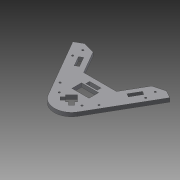
# Autodesk Inventor part: Frame_Upper_Plate_Bottom
Saved by Autodesk Inventor 2014 (Build 180170000, 170)
## iProperties
Created: 2014-08-25
Part Number: Frame_Upper_Plate_Bottom
Material: Generic
Document SubType Name: Modeling
Designer: ThatOtherGuy
Density: 1 g/cm^3
Appearance: Default
Author: ThatOtherGuy
Autodesk Inventor part; units mm, degrees
ref_plane "YZ Plane" through (0, 0, 0) normal (1, 0, 0) x (0, 1, 0)
ref_plane "XZ Plane" through (0, 0, 0) normal (0, 1, 0) x (-1, 0, 0)
ref_plane "XY Plane" through (0, 0, 0) normal (0, 0, 1) x (1, 0, 0)
sketch "Sketch1" plane through (0, 0, 0) normal (0, 0, 1) x (1, 0, 0)
  line L0 (-10.6066, 0) -> (0, 10.6066)
  line L1 (0, 10.6066) -> (10.6066, 0)
  line L2 (10.6066, 0) -> (0, -10.6066)
  line L3 (0, -10.6066) -> (-10.6066, 0)
  arc A0 (-25.9808, -15) -> (25.9808, -15) centre (0, 0) ccw
  line L4 (25.9808, -15) -> (85, 87.2243)
  line L5 (10, 41.731) -> (10, 35)
  line L6 (10, 35) -> (-10, 35)
  line L7 (-10, 35) -> (-10, 41.731)
  line L8 (-10, 41.731) -> (10, 41.731)
  line L9 (-85, 87.2243) -> (-25.9808, -15)
  circle A1 centre (-49.0748, 40) radius 1.6
  circle A2 centre (-64.0748, 65.9808) radius 1.6
  circle A3 centre (49.0748, 40) radius 1.6
  circle A4 centre (64.0748, 65.9808) radius 1.6
  line L10 (-85, 87.2243) -> (-72.0096, 94.7243)
  line L11 (-51.5192, 89.2339) -> (-28.8675, 50)
  line L12 (-28.8675, 50) -> (28.8675, 50)
  line L13 (28.8675, 50) -> (51.5192, 89.2339)
  line L14 (2.6517, -7.955) -> (7.955, -2.6517)
  line L15 (7.955, -2.6517) -> (12.7145, -7.4112)
  line L16 (12.7145, -7.4112) -> (7.4112, -12.7145)
  line L17 (7.4112, -12.7145) -> (2.6517, -7.955)
  line L18 (-2.6517, -7.955) -> (-7.4112, -12.7145)
  line L19 (-7.4112, -12.7145) -> (-12.7145, -7.4112)
  line L20 (-12.7145, -7.4112) -> (-7.955, -2.6517)
  line L21 (-7.955, -2.6517) -> (-2.6517, -7.955)
  circle A5 centre (-38.567, 40) radius 1.6
  circle A6 centre (38.567, 40) radius 1.6
  circle A7 centre (-63.567, 83.3013) radius 1.6
  circle A8 centre (63.567, 83.3013) radius 1.6
  circle A9 centre (-20, -1.6) radius 1.6
  circle A10 centre (20, -1.6) radius 1.6
  line L22 (-57.4526, 69.5109) -> (-47.4526, 52.1904)
  line L23 (-47.4526, 52.1904) -> (-41.6234, 55.5559)
  line L24 (-41.6234, 55.5559) -> (-51.6234, 72.8764)
  line L25 (-51.6234, 72.8764) -> (-57.4526, 69.5109)
  line L26 (47.4526, 52.1904) -> (57.4526, 69.5109)
  line L27 (57.4526, 69.5109) -> (51.6234, 72.8764)
  line L28 (51.6234, 72.8764) -> (41.6234, 55.5559)
  line L29 (41.6234, 55.5559) -> (47.4526, 52.1904)
  line L30 (-15, 32.5) -> (15, 32.5)
  line L31 (15, 32.5) -> (15, 15.6066)
  line L32 (15, 15.6066) -> (-15, 15.6066)
  line L33 (-15, 15.6066) -> (-15, 32.5)
  line L34 (-10.6066, 0) -> (10.6066, 0)
  line L35 (25.9808, -15) -> (0, -60)
  line L36 (0, -60) -> (-25.9808, -15)
  line L37 (85, 87.2243) -> (72.0096, 94.7243)
  circle A11 centre (-34.0748, 14.0192) radius 1.6
  circle A12 centre (34.0748, 14.0192) radius 1.6
  line L38 (72.0096, 94.7243) -> (51.5192, 89.2339)
  line L39 (-51.5192, 89.2339) -> (-72.0096, 94.7243)
  point P0 (0, 0)
  point P1 (0, 35)
  point P2 (0, 32.5)
  dimension "d0" = 15
  dimension "d9" = 30
  dimension "d11" = 6.731
  dimension "d12" = 20
  dimension "d25" = 60
  dimension "d34" = 3.2
  dimension "d36" = 30
  dimension "d38" = 30
  dimension "d40" = 7.5
  dimension "d41" = 7.5
  dimension "d42" = 7.5
  dimension "d43" = 7.5
  dimension "d45" = 40
  dimension "d54" = 50
  dimension "d55" = 0
  dimension "d56" = 0
  dimension "d57" = 7.5
  dimension "d58" = 3.75
  dimension "d63" = 15
  dimension "d64" = 3.2
  dimension "d66" = 50
  dimension "d67" = 15
  dimension "d68" = 15
  dimension "d73" = 20
  dimension "d74" = 15
  dimension "d75" = 15
  dimension "d76" = 15
  dimension "d77" = 15
  dimension "d79" = 35
  dimension "d80" = 2.5
  dimension "d81" = 5
  dimension "d82" = 30
  dimension "d83" = 20
  dimension "d84" = 20
  dimension "d85" = 40
  dimension "d86" = 170
  dimension "d88" = 30
  dimension "d89" = 30
  dimension "d90" = 7.5
  dimension "d91" = 7.5
  dimension "d92" = 135
  dimension "d93" = 30
  dimension "d94" = 45
  dimension "d95" = 15
  constraints: 80 end point, 14 parallel, 13 centre point, 13 equal length, 13 perpendicular, 10 equal radius, 7 horizontal alignment, 4 vertical alignment, 3 horizontal, 3 tangent, 2 collinear, 2 midpoint, 2 point on circle, 1 coincident
  measures "d0" distance of L0.start L0.end
  measures "d9" radius of A0
  measures "d11" distance of L5.start L5.end
  measures "d12" distance of L5.end L6.end
  measures "d25" angle of L9 L4
  measures "d34" diameter of A2
  measures "d36" distance of A1.centre A2.centre
  measures "d38" distance of A4.centre A3.centre
  measures "d40" distance from line of L4 A3.centre
  measures "d41" distance from line of L4 A4.centre
  measures "d42" distance from line of L9 A1.centre
  measures "d43" distance from line of L9 A2.centre
  measures "d45" vertical distance of A1.centre L0.start
  measures "d54" distance from line of point (0, 0) L12
  measures "d55" distance between parallel lines of L2 L14
  measures "d56" distance between parallel lines of L3 L21
  measures "d57" distance of L18.end L19.end
  measures "d58" distance between parallel lines of L2 L18
  measures "d63" distance edge to line of A6 L4
  measures "d64" diameter of A5
  measures "d66" distance of A5.centre A7.centre
  measures "d67" distance edge to line of A7 L9
  measures "d68" distance edge to line of A8 L4
  measures "d73" distance of L27.end L28.end
  measures "d74" distance between parallel lines of L4 L26
  measures "d75" distance between parallel lines of L9 L22
  measures "d76" distance edge to line of A5 L9
  measures "d77" distance from line of L23 A5.centre
  measures "d79" distance from line of point (0, 0) L6
  measures "d80" distance between parallel lines of L6 L30
  measures "d81" distance from line of L0.end L32
  measures "d82" distance of L30.start L30.end
  measures "d83" horizontal distance of A9.centre point (0, 0)
  measures "d84" horizontal distance of A10.centre point (0, 0)
  measures "d85" vertical distance of point (0, 0) A5.centre
  measures "d86" distance of L4.end L35.end
  measures "d88" distance of A11.centre A1.centre
  measures "d89" distance of A3.centre A12.centre
  measures "d90" distance from line of L9 A11.centre
  measures "d91" distance from line of L4 A12.centre
  measures "d92" angle of L10 L39
  measures "d93" distance between parallel lines of L11 L9
  measures "d94" angle of L37 L38
  measures "d95" distance of L9.start L10.end
extrude "Extrusion2" add sketch "Sketch1" along normal blind 6.731 contours L9 L10 L39 L11 L12 L13 L38 L37 L4 A0 | A5 | A6
sketch "Sketch2" plane through (0, 0, 6.731) normal (0, 0, 1) x (1, 0, 0)
  circle A0 centre (49.0748, 40) radius 1.6 projected
  circle A1 centre (-49.0748, 40) radius 1.6 projected
extrude "Extrusion3" add sketch "Sketch2" against normal up to surface (6.731 mm away)
equation "\"d38\" = d36"
equation "\"d41\" = d40"
equation "\"d58\" = 0.5 * d57"
equation "\"THICKA\" = 3.175"
equation "\"THICKB\" = 6.731"
equation "\"THICKC\" = 12.7"
equation "\"BALLDIA\" = 12"
equation "\"MAGDIA\" = 9.5"
equation "\"THICKPLY\" = 5"
body "Solid2"
